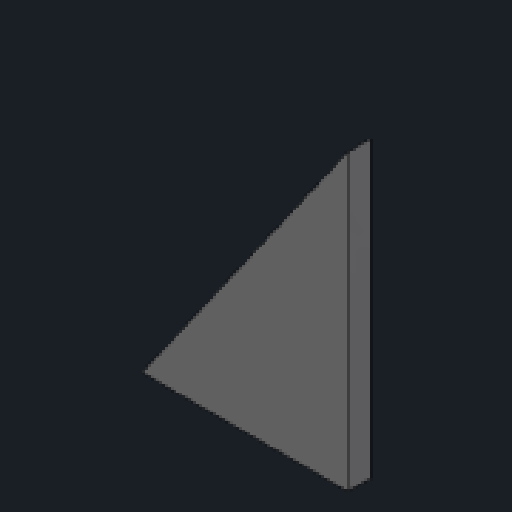
# Autodesk Inventor part: Front Hitch Model-2_Sheet Stifferner-2
Saved by Autodesk Inventor 2025.1 (Build 291241000, 241)
## iProperties
RuleStatus: InUse
Created: 2026-02-13
Part Number: Front Hitch Model-2_Sheet Stifferner-2
User Status: Released
Material: SS304
Document SubType Name: Sheet Metal
Designer: Desktop -24
Density: 7.99949 g/cm^3
Sheet Metal Rule: 3/8" (3.150 Die)
Appearance: Semi-Polished(1)
AfterDocNew0: Mat. Selection
encoded128: ÌSheet Metal (in)XÎ
Family: SS304
Author: Desktop -24
Revision Number: 0
Autodesk Inventor part; units mm, degrees
ref_plane "YZ Plane" through (0, 0, 0) normal (1, 0, 0) x (0, 1, 0)
ref_plane "XZ Plane" through (0, 0, 0) normal (0, 1, 0) x (-1, 0, 0)
ref_plane "XY Plane" through (0, 0, 0) normal (0, 0, 1) x (1, 0, 0)
sketch "Sketch1" plane through (0, 0, 0) normal (0, 0, 1) x (1, 0, 0)
  line L0 (0, 0) -> (-88.9, 0)
  line L1 (0, 0) -> (0, 127)
  line L2 (0, 127) -> (-88.9, 0)
  dimension "d29" = 88.9
  dimension "d30" = 127
  measures "d29" distance of L0.start L0.end
  measures "d30" distance of L0.start L1.end
extrude "Plate1" add sketch "Sketch1" along normal blind 9.525
equation "\"d15\" = Thickness"
equation "\"BendReliefWidth\" = Thickness"
equation "\"BendReliefDepth\" = 0.5 * Thickness"
equation "\"CornerReliefSize\" = 4 * Thickness"
equation "\"MinimumRemnant\" = 2 * Thickness"
equation "\"TransitionRadius\" = BendRadius"
equation "\"JacobiRadiusSize\" = Thickness"
equation "\"GapSize\" = Thickness"
equation "\"Thickness\" = 9.525"
equation "\"BendRadius\" = 13.208"
body "Solid1"
